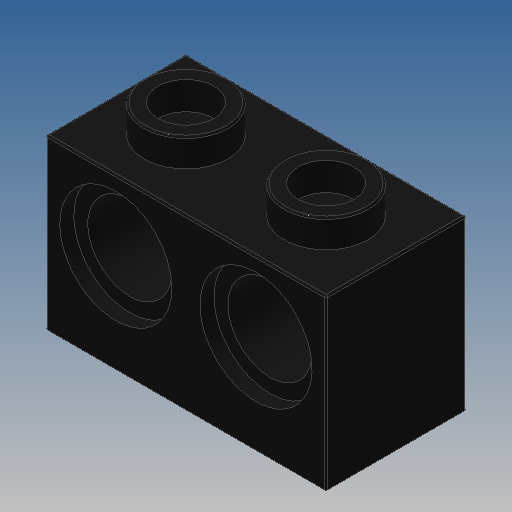
# Autodesk Inventor part: 32000-Black
Saved by Autodesk Inventor 2022.2 (Build 262287000, 287)
## iProperties
Created: 2014-06-03
Part Number: 32000-Black
Material: ABS Plastic
Document SubType Name: Modeling
Designer: D. Kohfeld
Density: 1.06 g/cm^3
Appearance: Black
Mass: 0.787366 g
Surface Area: 11.2832 cm^2
Volume: 0.742798 cm^3
Author: D. Kohfeld
Autodesk Inventor part; units mm, degrees
ref_plane "XZ Plane" through (0, 0, 0) normal (0, 1, 0) x (-1, 0, 0)
ref_plane "XY Plane" through (0, 0, 0) normal (0, 0, 1) x (1, 0, 0)
sketch "Sketch2" plane through (0, 0, 0) normal (0, 1, 0) x (-1, 0, 0)
  line L0 (-8, -4) -> (8, -4)
  line L1 (-8, 4) -> (8, 4)
  line L2 (-8, -4) -> (-8, 4)
  line L3 (8, 4) -> (8, -4)
  point P0 (0, 0)
  point P1 (0, 4)
  point P2 (-8, 0)
  dimension "d58" = 16
  dimension "d59" = 8
  constraints: 8 end point, 2 horizontal, 2 midpoint, 2 parallel, 1 horizontal alignment, 1 perpendicular, 1 vertical alignment
  measures "d58" distance of L0.start L0.end
  measures "d59" distance between parallel lines of L0 L1
extrude "Extrusion1" add sketch "Sketch2" along normal blind 9.6
sketch "Sketch9" plane through (0, 0, 0) normal (0, -1, 0) x (1, 0, 0)
  line L0 (-8, 4) -> (8, 4) projected
  line L1 (-8, -4) -> (-8, 4) projected
  line L2 (-6.5, 2.5) -> (6.5, 2.5)
  line L3 (6.5, 2.5) -> (6.5, -2.5)
  line L4 (6.5, -2.5) -> (-6.5, -2.5)
  line L5 (-6.5, -2.5) -> (-6.5, 2.5)
  point P0 (0, 0)
  point P1 (0, 2.5)
  point P2 (-6.5, 0)
  dimension "d61" = 1.5
  dimension "d62" = 1.5
  constraints: 8 end point, 2 midpoint, 2 parallel, 1 horizontal, 1 horizontal alignment, 1 perpendicular, 1 vertical alignment
  measures "d61" distance between parallel lines of L1 L5
  measures "d62" distance between parallel lines of L0 L2
extrude "Extrusion4" cut sketch "Sketch9" against normal blind 8
sketch "Sketch11" plane through (-8, 0, 4) normal (0, 0, 1) x (1, 0, 0)
  line L0 (0, 0) -> (16, 0) projected
  line L1 (0, 9.6) -> (16, 9.6) projected
  line L2 (0, 0) -> (0, 9.6) projected
  line L3 (7.6, 8) -> (0.4, 8)
  line L4 (0.4, 8) -> (0.4, 5.6)
  arc A0 (0.4, 5.6) -> (7.6, 5.6) centre (4, 5.6) ccw
  line L5 (7.6, 5.6) -> (7.6, 8)
  point P0 (8, 0)
  point P1 (8, 9.6)
  dimension "d93" = 1.6
  dimension "d94" = 4
  dimension "d96" = 7.2
  dimension "d97" = 5.6
  constraints: 6 end point, 2 perpendicular, 2 point on circle, 2 tangent, 1 centre point, 1 midpoint, 1 parallel
  measures "d93" distance between parallel lines of L1 L3
  measures "d94" horizontal distance of A0.centre point (8, 9.6)
  measures "d96" diameter of A0
  measures "d97" distance from line of A0.centre L0
extrude "Extrusion5" add sketch "Sketch11" against normal blind 8
sketch "Sketch4" plane through (0, 9.6, 0) normal (0, 1, 0) x (1, 0, 0)
  circle A0 centre (-4, 0) radius 2.4
  circle A1 centre (-4, 0) radius 1.6
  line L0 (-8, 4) -> (-8, -4) projected
  point P0 (-8, 0)
  dimension "d13" = 4.8
  dimension "d57" = 3.2
  dimension "d69" = 4
  constraints: 2 centre point, 1 coincident, 1 horizontal alignment, 1 midpoint
  measures "d13" diameter of A0
  measures "d57" diameter of A1
  measures "d69" distance from line of A0.centre L0
extrude "Extrusion3" add sketch "Sketch4" along normal blind 1.6
sketch3d "Sketch12"
  constraints: 50 end point, 41 tangent, 38 point on circle, 19 centre point, 14 parallel, 13 equal radius, 10 horizontal, 4 collinear, 4 concentric, 3 point on line, 1 coincident, 1 midpoint, 1 other
feature "LEGO_SM:1" [suppressed]
fillet "Fillet1" radius 0.1 1 edges at (-6.4, 11.2, 0)
pattern_linear "Rectangular Pattern2" count 2 spacing 8 along (1, 0, 0) of "Extrusion3", "Fillet1", "Extrusion5"
fillet "Fillet2" radius 0.1 8 edges at (-8, 9.6, 0) (-8, 4.8, 4) (0, 9.6, 4) (-8, 4.8, -4) (0, 9.6, -4) (8, 4.8, 4) (8, 9.6, 0) (8, 4.8, -4)
ref_plane "Work Plane1" through (-4, 0, 0) normal (1, 0, 0) x (0, 1, 0)
sketch "Sketch10" plane through (-4, 0, 0) normal (1, 0, 0) x (0, 1, 0)
  line L0 (0, -3.9) -> (0, 3.9) projected
  line L1 (0, 4) -> (9.5, 4) projected
  line L2 (9.5, -4) -> (0, -4) projected
  line L3 (5.6, 4) -> (5.6, -4)
  line L4 (5.6, -4) -> (8.8, -4)
  line L5 (8.8, -4) -> (8.8, -3.2)
  line L6 (8.8, -3.2) -> (8, -3.2)
  line L7 (8, -3.2) -> (8, 3.2)
  line L8 (8, 3.2) -> (8.8, 3.2)
  line L9 (8.8, 3.2) -> (8.8, 4)
  line L10 (8.8, 4) -> (5.6, 4)
  line L11 (8.8, 4) -> (9.5, 4)
  line L12 (9.5, -4) -> (8.8, -4)
  line L13 (9.5, -4) -> (9.5, 4)
  point P0 (0, 0)
  dimension "d75" = 5.6
  dimension "d76" = 0.8
  dimension "d77" = 4.8
  dimension "d78" = 6.4
  constraints: 22 end point, 6 perpendicular, 4 point on line, 2 collinear, 2 equal length, 2 parallel
  measures "d75" distance between parallel lines of L3 L0
  measures "d76" distance of L8.end L9.end
  measures "d77" diameter of L7 L3
  measures "d78" diameter of L9 L3
revolve "Revolution1" cut sketch "Sketch10" angle 360 about axis through (-4, 5.6, 4) along (0, 0, -1) contours L1 L9 L8 L7 L6 L5 L2 L3
pattern_linear "Rectangular Pattern4" count 2 spacing 8 along (1, 0, 0) of "Revolution1"
equation "\"d58\" = 8 * knobs"
equation "\"d4\" = lh"
equation "\"d62\" = d61"
equation "\"d63\" = bd"
equation "\"d93\" = topthk"
equation "\"d94\" = 0.5 * lu"
equation "\"d96\" = tlad"
equation "\"d97\" = th"
equation "\"d13\" = kd"
equation "\"d57\" = rd"
equation "\"d69\" = 0.5 * lu"
equation "\"d20\" = knobh"
equation "\"d72\" = lu"
equation "\"d75\" = th"
equation "\"d76\" = tsl"
equation "\"d77\" = tpd"
equation "\"d78\" = tsd"
equation "\"d89\" = -0.5 * lu"
equation "\"knobs\" = 2"
equation "\"lh\" = 9.6"
equation "\"bd\" = 8"
equation "\"topthk\" = 1.6"
equation "\"tlad\" = 7.2"
equation "\"th\" = 5.6"
equation "\"kd\" = 4.8"
equation "\"rd\" = 3.2"
equation "\"lu\" = 8"
equation "\"knobh\" = 1.6"
equation "\"tsl\" = 0.8"
equation "\"tpd\" = 4.8"
equation "\"tsd\" = 6.4"
body "Solid1"
